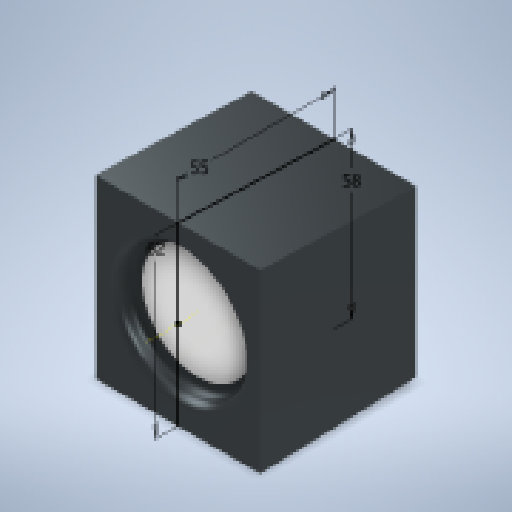
# Autodesk Inventor part: Колонка
Saved by Autodesk Inventor 2023.2 (Build 272271030, 271C)
## iProperties
Created: 2024-03-25
Part Number: Колонка
Material: Типовые
Document SubType Name: Modeling
Designer: I9232
Density: 1 g/cm^3
Appearance: Чугун серый
Author: I9232
Autodesk Inventor part; units mm, degrees
ref_plane "YZ Plane" through (0, 0, 0) normal (1, 0, 0) x (0, 1, 0)
ref_plane "XZ Plane" through (0, 0, 0) normal (0, 1, 0) x (-1, 0, 0)
ref_plane "XY Plane" through (0, 0, 0) normal (0, 0, 1) x (1, 0, 0)
sketch "Эскиз1" plane through (0, 0, 0) normal (1, 0, 0) x (0, 1, 0)
  line L0 (31, 28.4167) -> (-31, 28.4167)
  line L1 (29, -26.5833) -> (-29, -26.5833)
  line L2 (-29, -26.5833) -> (-31, 28.4167)
  line L3 (29, -26.5833) -> (31, 28.4167)
  line L4 (29, -26.5833) -> (-31, 28.4167) construction
  line L5 (31, 28.4167) -> (-29, -26.5833) construction
  line L6 (0, 39.4167) -> (0, -37.5833) construction
  point P0 (0, 0)
  point P1 (0, 0)
  point P2 (0, 0)
  point P3 (0, 28.4167)
  dimension "d0" = 58
  dimension "d1" = 62
  dimension "d2" = 55
  constraints: 12 end point, 3 point on line, 2 coincident, 2 horizontal, 1 midpoint
  measures "d0" distance of L1.start L1.end
  measures "d1" distance of L0.start L0.end
  measures "d2" vertical distance of L1.start L0.start
extrude "Выдавливание1" add sketch "Эскиз1" along normal mid plane 58
sketch "Эскиз2" plane through (-29, -31, 28.4167) normal (0, 0, 1) x (1, 0, 0)
  circle A0 centre (29, 31) radius 22.5
  dimension "d5" = 45
  constraints: 1 centre point, 1 coincident
  measures "d5" diameter of A0
extrude "Выдавливание2" cut sketch "Эскиз2" against normal blind 7
fillet "Сопряжение1" radius 3 2 edges at (-22.5, 0, 21.4167) (-22.5, 0, 28.4167)
sketch "Эскиз4" plane through (29, 29, -26.5833) normal (0, 0, -1) x (-1, 0, 0)
  circle A0 centre (7.95, -7.95) radius 1.5
  circle A1 centre (7.95, -50.05) radius 1.5
  circle A2 centre (50.05, -50.05) radius 1.5
  circle A3 centre (50.05, -7.95) radius 1.5
  line L0 (0, -58) -> (0, 0) projected
  line L1 (58, 0) -> (0, 0) projected
  line L2 (29, -21.9997) -> (29, -36.0003) construction
  line L3 (24.7856, -29) -> (33.2144, -29) construction
  line L4 (33.2144, -29) -> (24.7856, -29) construction
  line L5 (7.95, -7.95) -> (50.05, -7.95) construction
  line L6 (50.05, -7.95) -> (50.05, -50.05) construction
  line L7 (50.05, -50.05) -> (7.95, -50.05) construction
  line L8 (7.95, -7.95) -> (7.95, -50.05) construction
  line L9 (7.95, -7.95) -> (50.05, -50.05) construction
  line L10 (7.95, -50.05) -> (50.05, -7.95) construction
  point P0 (29, -29)
  point P1 (29, -29)
  point P2 (29, -29)
  dimension "d15" = 3
  dimension "d24" = 42.1
  constraints: 18 end point, 4 centre point, 4 midpoint, 3 equal length, 3 equal radius, 2 coincident, 2 perpendicular, 2 symmetric about line, 2 vertical, 1 horizontal
  measures "d15" diameter of A2
  measures "d24" distance of L5.start L7.end
extrude "Выдавливание5" cut sketch "Эскиз4" against normal blind 10
